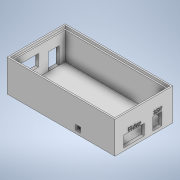
# Autodesk Inventor part: Caixa plaquinha valvula
Saved by Autodesk Inventor 2020 (Build 240168000, 168)
## iProperties
Created: 2022-10-16
Part Number: Caixa plaquinha valvula
Material: Genérico
Document SubType Name: Modeling
Designer: Gabriel
Density: 1 g/cm^3
Appearance: Padrão
Author: Gabriel
Autodesk Inventor part; units mm, degrees
ref_plane "YZ Plane" through (0, 0, 0) normal (1, 0, 0) x (0, 1, 0)
ref_plane "XZ Plane" through (0, 0, 0) normal (0, 1, 0) x (-1, 0, 0)
ref_plane "XY Plane" through (0, 0, 0) normal (0, 0, 1) x (1, 0, 0)
sketch "Esboço1" plane through (0, 0, 0) normal (0, 1, 0) x (-1, 0, 0)
  line L0 (62.5795, 27.2159) -> (-45.4205, 27.2159)
  line L1 (-45.4205, 27.2159) -> (-45.4205, -30.7841)
  line L2 (-45.4205, -30.7841) -> (62.5795, -30.7841)
  line L3 (62.5795, -30.7841) -> (62.5795, 27.2159)
  point P0 (0, 0)
  dimension "d0" = 58
  dimension "d1" = 108
  constraints: 8 end point, 2 parallel, 1 horizontal, 1 perpendicular
  measures "d0" distance between parallel lines of L2 L0
  measures "d1" distance of L1.end L2.end
extrude "Extrusão1" add sketch "Esboço1" along normal blind 32
sketch "Esboço2" plane through (0, 32, 0) normal (0, 1, 0) x (1, 0, 0)
  line L0 (-59.5795, 27.7841) -> (42.4205, 27.7841)
  line L1 (42.4205, 27.7841) -> (42.4205, -24.2159)
  line L2 (42.4205, -24.2159) -> (-59.5795, -24.2159)
  line L3 (-59.5795, -24.2159) -> (-59.5795, 27.7841)
  line L4 (-62.5795, 30.7841) -> (-62.5795, -27.2159) projected
  line L5 (45.4205, 30.7841) -> (-62.5795, 30.7841) projected
  point P0 (0, 0)
  dimension "d4" = 3
  dimension "d5" = 102
  dimension "d6" = 3
  dimension "d7" = 52
  constraints: 8 end point, 2 parallel, 1 horizontal, 1 perpendicular
  measures "d4" distance between parallel lines of L4 L3
  measures "d5" distance between parallel lines of L1 L3
  measures "d6" distance between parallel lines of L5 L0
  measures "d7" distance between parallel lines of L0 L2
extrude "Extrusão2" cut sketch "Esboço2" against normal blind 30
sketch "Esboço4" plane through (0, 32, 0) normal (0, 1, 0) x (1, 0, 0)
  line L0 (-61.0795, 29.2841) -> (43.9205, 29.2841)
  line L1 (43.9205, 29.2841) -> (43.9205, -25.7159)
  line L2 (43.9205, -25.7159) -> (-61.0795, -25.7159)
  line L3 (-61.0795, -25.7159) -> (-61.0795, 29.2841)
  line L4 (45.4205, 30.7841) -> (-62.5795, 30.7841) projected
  line L5 (-62.5795, 30.7841) -> (-62.5795, -27.2159) projected
  line L6 (-62.5795, -27.2159) -> (45.4205, -27.2159) projected
  line L7 (45.4205, -27.2159) -> (45.4205, 30.7841) projected
  point P0 (0, 0)
  dimension "d10" = 1.5
  dimension "d11" = 1.5
  dimension "d12" = 1.5
  dimension "d13" = 1.5
  constraints: 8 end point, 2 parallel, 1 horizontal, 1 perpendicular
  measures "d10" distance between parallel lines of L4 L0
  measures "d11" distance between parallel lines of L5 L3
  measures "d12" distance between parallel lines of L6 L2
  measures "d13" distance between parallel lines of L7 L1
extrude "Extrusão3" cut sketch "Esboço4" against normal blind 2.5 contours L0 L1 L2 L3
sketch "Esboço5" plane through (42.4205, 2, -27.7841) normal (-1, 0, 0) x (0, 0, 1)
  line L0 (0, 0) -> (52, 0) projected
  line L1 (8.1, 0) -> (17.1, 0)
  line L2 (17.1, 0) -> (17.1, 13.5)
  line L3 (17.1, 13.5) -> (8.1, 13.5)
  line L4 (8.1, 13.5) -> (8.1, 0)
  line L5 (46.3, 0) -> (25.6, 0)
  line L6 (25.6, 0) -> (25.6, 12)
  line L7 (25.6, 12) -> (46.3, 12)
  line L8 (46.3, 12) -> (46.3, 0)
  line L9 (52, 27.5) -> (0, 27.5) projected
  point P0 (27.7841, -2)
  point P1 (25.6, 0)
  point P2 (17.1, 0)
  dimension "d17" = 9
  dimension "d18" = 13.5
  dimension "d20" = 20.7
  dimension "d21" = 12
  dimension "d23" = 8.5
  dimension "d24" = 8.1
  dimension "d25" = 5.7
  dimension "d28" = 15.5
  constraints: 16 end point, 4 parallel, 2 horizontal, 2 perpendicular, 2 point on line
  measures "d17" distance between parallel lines of L2 L4
  measures "d18" distance between parallel lines of L0 L3
  measures "d20" distance between parallel lines of L6 L8
  measures "d21" distance between parallel lines of L0 L7
  measures "d23" distance between parallel lines of L6 L2
  measures "d24" distance from line of L9.end L4
  measures "d25" distance from line of L9.start L8
  measures "d28" distance between parallel lines of L9 L7
extrude "Extrusão4" cut sketch "Esboço5" against normal blind 5
sketch "Esboço6" plane through (0, 2, 0) normal (0, 1, 0) x (1, 0, 0)
  line L0 (45.4205, 2.1841) -> (45.4205, -18.5159) projected
  line L1 (42.4205, 10.6841) -> (42.4205, 2.1841) projected
  line L2 (45.4205, -18.5159) -> (42.4205, -18.5159)
  line L3 (42.4205, -18.5159) -> (42.4205, 2.1841)
  line L4 (42.4205, 2.1841) -> (45.4205, 2.1841)
  line L5 (45.4205, 2.1841) -> (45.4205, -18.5159)
  line L6 (45.4205, 19.6841) -> (45.4205, 10.6841) projected
  line L7 (45.4205, 19.6841) -> (42.4205, 19.6841)
  line L8 (42.4205, 19.6841) -> (42.4205, 10.6841)
  line L9 (42.4205, 10.6841) -> (45.4205, 10.6841)
  line L10 (45.4205, 10.6841) -> (45.4205, 19.6841)
  point P0 (0, 0)
  constraints: 16 end point, 4 parallel, 2 horizontal, 2 perpendicular, 1 point on line
extrude "Extrusão5" add sketch "Esboço6" along normal blind 1
sketch "Esboço7" plane through (-59.5795, 2, 24.2159) normal (1, 0, 0) x (0, 0, -1)
  line L0 (46, 0.1025) -> (35, 0.1025)
  line L1 (35, 0.1025) -> (35, 17.0506)
  line L2 (35, 17.0506) -> (46, 17.0506)
  line L3 (46, 17.0506) -> (46, 0.1025)
  line L4 (3.908, 8.6) -> (25.408, 8.6)
  line L5 (25.408, 8.6) -> (25.408, 20.6)
  line L6 (25.408, 20.6) -> (3.908, 20.6)
  line L7 (3.908, 20.6) -> (3.908, 8.6)
  line L8 (0, 0) -> (52, 0) projected
  point P0 (24.2159, -2)
  point P1 (52, 27.5)
  point P2 (0, 27.5)
  dimension "d31" = 6
  dimension "d32" = 11
  dimension "d33" = 3.908
  dimension "d34" = 21.5
  dimension "d35" = 12
  dimension "d36" = 8.6
  dimension "d39" = 16.948
  constraints: 16 end point, 4 parallel, 2 horizontal, 2 perpendicular
  measures "d31" distance from line of L3 point (52, 27.5)
  measures "d32" distance between parallel lines of L3 L1
  measures "d33" distance from line of point (0, 27.5) L7
  measures "d34" distance between parallel lines of L5 L7
  measures "d35" distance between parallel lines of L6 L4
  measures "d36" distance between parallel lines of L8 L4
  measures "d39" distance between parallel lines of L0 L2
extrude "Extrusão6" cut sketch "Esboço7" against normal blind 5
sketch "Esboço8" plane through (42.4205, 2, 24.2159) normal (0, 0, -1) x (-1, 0, 0)
  line L0 (0, 0) -> (102, 0) projected
  line L1 (36.5, 0) -> (31.5, 0)
  line L2 (31.5, 0) -> (31.5, 6)
  line L3 (31.5, 6) -> (36.5, 6)
  line L4 (36.5, 6) -> (36.5, 0)
  line L5 (0, 27.5) -> (0, 0) projected
  point P0 (42.4205, -2)
  dimension "d41" = 5
  dimension "d43" = 31.5
  dimension "d44" = 6
  dimension "d45" = 6
  constraints: 8 end point, 2 parallel, 1 horizontal, 1 perpendicular, 1 point on line
  measures "d41" distance between parallel lines of L4 L2
  measures "d43" distance between parallel lines of L5 L2
  measures "d44" distance between parallel lines of L3 L1
  measures "d45" distance between parallel lines of L0 L3
extrude "Extrusão7" cut sketch "Esboço8" against normal blind 5
sketch "Esboço9" plane through (0, 2, 0) normal (0, 1, 0) x (1, 0, 0)
  line L0 (5.9205, -24.2159) -> (-59.5795, -24.2159) projected
  line L1 (5.9205, -24.2159) -> (10.9205, -24.2159)
  line L2 (10.9205, -24.2159) -> (10.9205, -27.2159)
  line L3 (10.9205, -27.2159) -> (5.9205, -27.2159)
  line L4 (5.9205, -27.2159) -> (5.9205, -24.2159)
  line L5 (10.9205, -27.2159) -> (5.9205, -27.2159) projected
  point P0 (0, 0)
  dimension "d50" = 0
  constraints: 8 end point, 2 parallel, 1 horizontal, 1 perpendicular
  measures "d50" distance between parallel lines of L5 L3
extrude "Extrusão8" add sketch "Esboço9" along normal blind 1
sketch "Esboço10" plane through (45.4205, 0, 27.2159) normal (1, 0, 0) x (0, 0, -1)
  line L0 (36.0799, 21.9524) -> (48.8276, 21.9524) construction
  line L1 (48.8276, 21.9524) -> (48.8276, 15.4026) construction
  line L2 (48.8276, 15.4026) -> (36.0799, 15.4026) construction
  line L3 (36.0799, 15.4026) -> (36.0799, 21.9524) construction
  line L4 (13.7499, 18.2381) -> (24.4451, 18.2381) construction
  line L5 (24.4451, 18.2381) -> (24.4451, 15.1259) construction
  line L6 (24.4451, 15.1259) -> (13.7499, 15.1259) construction
  line L7 (13.7499, 15.1259) -> (13.7499, 18.2381) construction
  line L8 (16.286, 15.1881) -> (15.5247, 15.1881)
  line L9 (15.5247, 15.1881) -> (15.5247, 17.2099)
  line L10 (15.5247, 17.2099) -> (14.9711, 15.9049)
  line L11 (14.9711, 15.9049) -> (14.4471, 15.9049)
  line L12 (14.4471, 15.9049) -> (13.8935, 17.2099)
  line L13 (13.8935, 17.2099) -> (13.8935, 15.1881)
  line L14 (13.8935, 15.1881) -> (13.1717, 15.1881)
  line L15 (13.1717, 15.1881) -> (13.1717, 18.2381)
  line L16 (13.1717, 18.2381) -> (14.0541, 18.2381)
  line L17 (14.0541, 18.2381) -> (14.7313, 16.7329)
  line L18 (14.7313, 16.7329) -> (15.4036, 18.2381)
  line L19 (15.4036, 18.2381) -> (16.286, 18.2381)
  line L20 (16.286, 18.2381) -> (16.286, 15.1881)
  spline S0 degree 2 poles (19.0839, 16.3374) (19.0839, 15.769) (18.4635, 15.1165) (17.8975, 15.1165) knots 0 0 0 1 2 2 2
  spline S1 degree 2 poles (17.8975, 15.1165) (17.334, 15.1165) (16.7087, 15.769) (16.7087, 16.3374) knots 0 0 0 1 2 2 2
  spline S2 degree 2 poles (16.7087, 16.3374) (16.7087, 16.9109) (17.334, 17.5609) (17.8975, 17.5609) knots 0 0 0 1 2 2 2
  spline S3 degree 2 poles (17.8975, 17.5609) (18.461, 17.5609) (19.0839, 16.9084) (19.0839, 16.3374) knots 0 0 0 1 2 2 2
  spline S4 degree 2 poles (18.3498, 16.3325) (18.3498, 16.5376) (18.2831, 16.812) (18.2238, 16.8936) knots 0 0 0 1 2 2 2
  spline S5 degree 2 poles (18.2238, 16.8936) (18.1595, 16.9801) (17.9989, 17.0468) (17.8975, 17.0468) knots 0 0 0 1 2 2 2
  spline S6 degree 2 poles (17.8975, 17.0468) (17.7986, 17.0468) (17.6429, 16.9875) (17.5787, 16.9034) knots 0 0 0 1 2 2 2
  spline S7 degree 2 poles (17.5787, 16.9034) (17.5169, 16.8244) (17.4427, 16.5451) (17.4427, 16.3325) knots 0 0 0 1 2 2 2
  spline S8 degree 2 poles (17.4427, 16.3325) (17.4427, 16.1224) (17.5119, 15.8629) (17.5688, 15.7838) knots 0 0 0 1 2 2 2
  spline S9 degree 2 poles (17.5688, 15.7838) (17.6256, 15.7047) (17.7986, 15.6306) (17.9025, 15.6306) knots 0 0 0 1 2 2 2
  spline S10 degree 2 poles (17.9025, 15.6306) (17.989, 15.6306) (18.1669, 15.7047) (18.2213, 15.7789) knots 0 0 0 1 2 2 2
  spline S11 degree 2 poles (18.2213, 15.7789) (18.2831, 15.8654) (18.3498, 16.115) (18.3498, 16.3325) knots 0 0 0 1 2 2 2
  spline S12 degree 2 poles (20.3444, 15.1436) (19.907, 15.1436) (19.5065, 15.5045) (19.5065, 15.9148) knots 0 0 0 1 2 2 2
  line L21 (19.5065, 15.9148) -> (19.5065, 16.99)
  line L22 (19.5065, 16.99) -> (19.2322, 16.99)
  line L23 (19.2322, 16.99) -> (19.2322, 17.4892)
  line L24 (19.2322, 17.4892) -> (19.5065, 17.4892)
  line L25 (19.5065, 17.4892) -> (19.5065, 18.1467)
  line L26 (19.5065, 18.1467) -> (20.2233, 18.1467)
  line L27 (20.2233, 18.1467) -> (20.2233, 17.4892)
  line L28 (20.2233, 17.4892) -> (20.9154, 17.4892)
  line L29 (20.9154, 17.4892) -> (20.9154, 16.99)
  line L30 (20.9154, 16.99) -> (20.2233, 16.99)
  line L31 (20.2233, 16.99) -> (20.2233, 16.1718)
  spline S13 degree 2 poles (20.2233, 16.1718) (20.2233, 16.0507) (20.2283, 15.8703) (20.2579, 15.7986) knots 0 0 0 1 2 2 2
  spline S14 degree 2 poles (20.2579, 15.7986) (20.2876, 15.7269) (20.4334, 15.6429) (20.5718, 15.6429) knots 0 0 0 1 2 2 2
  spline S15 degree 2 poles (20.5718, 15.6429) (20.6311, 15.6429) (20.8165, 15.6923) (20.8536, 15.7121) knots 0 0 0 1 2 2 2
  line L32 (20.8536, 15.7121) -> (20.9154, 15.7121)
  line L33 (20.9154, 15.7121) -> (20.9154, 15.2079)
  spline S16 degree 2 poles (20.9154, 15.2079) (20.7992, 15.1782) (20.5372, 15.1436) (20.3444, 15.1436) knots 0 0 0 1 2 2 2
  spline S17 degree 2 poles (23.4142, 16.3374) (23.4142, 15.769) (22.7938, 15.1165) (22.2278, 15.1165) knots 0 0 0 1 2 2 2
  spline S18 degree 2 poles (22.2278, 15.1165) (21.6643, 15.1165) (21.039, 15.769) (21.039, 16.3374) knots 0 0 0 1 2 2 2
  spline S19 degree 2 poles (21.039, 16.3374) (21.039, 16.9109) (21.6643, 17.5609) (22.2278, 17.5609) knots 0 0 0 1 2 2 2
  spline S20 degree 2 poles (22.2278, 17.5609) (22.7914, 17.5609) (23.4142, 16.9084) (23.4142, 16.3374) knots 0 0 0 1 2 2 2
  spline S21 degree 2 poles (22.6801, 16.3325) (22.6801, 16.5376) (22.6134, 16.812) (22.5541, 16.8936) knots 0 0 0 1 2 2 2
  spline S22 degree 2 poles (22.5541, 16.8936) (22.4898, 16.9801) (22.3292, 17.0468) (22.2278, 17.0468) knots 0 0 0 1 2 2 2
  spline S23 degree 2 poles (22.2278, 17.0468) (22.129, 17.0468) (21.9732, 16.9875) (21.909, 16.9034) knots 0 0 0 1 2 2 2
  spline S24 degree 2 poles (21.909, 16.9034) (21.8472, 16.8244) (21.773, 16.5451) (21.773, 16.3325) knots 0 0 0 1 2 2 2
  spline S25 degree 2 poles (21.773, 16.3325) (21.773, 16.1224) (21.8422, 15.8629) (21.8991, 15.7838) knots 0 0 0 1 2 2 2
  spline S26 degree 2 poles (21.8991, 15.7838) (21.9559, 15.7047) (22.129, 15.6306) (22.2328, 15.6306) knots 0 0 0 1 2 2 2
  spline S27 degree 2 poles (22.2328, 15.6306) (22.3193, 15.6306) (22.4972, 15.7047) (22.5516, 15.7789) knots 0 0 0 1 2 2 2
  spline S28 degree 2 poles (22.5516, 15.7789) (22.6134, 15.8654) (22.6801, 16.115) (22.6801, 16.3325) knots 0 0 0 1 2 2 2
  line L34 (25.3396, 16.8095) -> (25.2803, 16.8095)
  spline S29 degree 2 poles (25.2803, 16.8095) (25.2383, 16.8244) (25.0826, 16.8392) (24.9886, 16.8392) knots 0 0 0 1 2 2 2
  spline S30 degree 2 poles (24.9886, 16.8392) (24.8774, 16.8392) (24.6278, 16.7725) (24.5116, 16.728) knots 0 0 0 1 2 2 2
  line L35 (24.5116, 16.728) -> (24.5116, 15.1881)
  line L36 (24.5116, 15.1881) -> (23.7948, 15.1881)
  line L37 (23.7948, 15.1881) -> (23.7948, 17.4892)
  line L38 (23.7948, 17.4892) -> (24.5116, 17.4892)
  line L39 (24.5116, 17.4892) -> (24.5116, 17.158)
  spline S31 degree 2 poles (24.5116, 17.158) (24.561, 17.2025) (24.7341, 17.3409) (24.8057, 17.3829) knots 0 0 0 1 2 2 2
  spline S32 degree 2 poles (24.8057, 17.3829) (24.8848, 17.4299) (25.0924, 17.4966) (25.1839, 17.4966) knots 0 0 0 1 2 2 2
  spline S33 degree 2 poles (25.1839, 17.4966) (25.2185, 17.4966) (25.305, 17.4917) (25.3396, 17.4892) knots 0 0 0 1 2 2 2
  line L40 (25.3396, 17.4892) -> (25.3396, 16.8095)
  line L41 (40.7496, 17.1229) -> (38.7352, 17.1229)
  line L42 (38.7352, 17.1229) -> (38.7352, 17.6543)
  line L43 (38.7352, 17.6543) -> (39.3778, 17.6543)
  line L44 (39.3778, 17.6543) -> (39.3778, 19.2683)
  line L45 (39.3778, 19.2683) -> (38.7352, 19.2683)
  line L46 (38.7352, 19.2683) -> (38.7352, 19.7651)
  spline S34 degree 2 poles (38.7352, 19.7651) (38.8761, 19.7651) (39.1554, 19.8021) (39.2394, 19.8417) knots 0 0 0 1 2 2 2
  spline S35 degree 2 poles (39.2394, 19.8417) (39.3358, 19.8911) (39.4445, 20.0567) (39.4544, 20.1803) knots 0 0 0 1 2 2 2
  line L47 (39.4544, 20.1803) -> (40.1218, 20.1803)
  line L48 (40.1218, 20.1803) -> (40.1218, 17.6543)
  line L49 (40.1218, 17.6543) -> (40.7496, 17.6543)
  line L50 (40.7496, 17.6543) -> (40.7496, 17.1229)
  line L51 (43.5573, 17.1229) -> (41.3156, 17.1229)
  line L52 (41.3156, 17.1229) -> (41.3156, 17.6197)
  spline S36 degree 2 poles (41.3156, 17.6197) (41.5998, 17.8471) (42.0546, 18.2475) (42.2251, 18.4279) knots 0 0 0 1 2 2 2
  spline S37 degree 2 poles (42.2251, 18.4279) (42.45, 18.6627) (42.6502, 19.0211) (42.6502, 19.2089) knots 0 0 0 1 2 2 2
  spline S38 degree 2 poles (42.6502, 19.2089) (42.6502, 19.4215) (42.3957, 19.6489) (42.1683, 19.6489) knots 0 0 0 1 2 2 2
  spline S39 degree 2 poles (42.1683, 19.6489) (42.0521, 19.6489) (41.8445, 19.592) (41.7382, 19.5476) knots 0 0 0 1 2 2 2
  spline S40 degree 2 poles (41.7382, 19.5476) (41.6344, 19.5006) (41.4861, 19.4017) (41.449, 19.377) knots 0 0 0 1 2 2 2
  line L53 (41.449, 19.377) -> (41.3897, 19.377)
  line L54 (41.3897, 19.377) -> (41.3897, 20.0419)
  spline S41 degree 2 poles (41.3897, 20.0419) (41.5182, 20.1037) (42.0669, 20.2322) (42.3215, 20.2322) knots 0 0 0 1 2 2 2
  spline S42 degree 2 poles (42.3215, 20.2322) (42.8653, 20.2322) (43.4239, 19.7478) (43.4239, 19.3103) knots 0 0 0 1 2 2 2
  spline S43 degree 2 poles (43.4239, 19.3103) (43.4239, 19.0409) (43.1693, 18.5218) (42.8752, 18.2252) knots 0 0 0 1 2 2 2
  spline S44 degree 2 poles (42.8752, 18.2252) (42.6898, 18.0423) (42.3413, 17.7581) (42.2647, 17.6988) knots 0 0 0 1 2 2 2
  line L55 (42.2647, 17.6988) -> (43.5573, 17.6988)
  line L56 (43.5573, 17.6988) -> (43.5573, 17.1229)
  line L57 (46.5406, 20.1729) -> (45.4926, 17.1229)
  line L58 (45.4926, 17.1229) -> (44.6943, 17.1229)
  line L59 (44.6943, 17.1229) -> (43.6463, 20.1729)
  line L60 (43.6463, 20.1729) -> (44.4397, 20.1729)
  line L61 (44.4397, 20.1729) -> (45.1046, 18.1041)
  line L62 (45.1046, 18.1041) -> (45.767, 20.1729)
  line L63 (45.767, 20.1729) -> (46.5406, 20.1729)
  point P0 (27.2159, 0)
  constraints: 4 other
extrude "Extrusão9" add sketch "Esboço10" along normal blind 0.8
sketch "Esboço11" plane through (-62.5795, 0, -30.7841) normal (-1, 0, 0) x (0, 0, 1)
  line L0 (35.5434, 8.3072) -> (44.2454, 8.3072) construction
  line L1 (44.2454, 8.3072) -> (44.2454, 5.1577) construction
  line L2 (44.2454, 5.1577) -> (35.5434, 5.1577) construction
  line L3 (35.5434, 5.1577) -> (35.5434, 8.3072) construction
  line L4 (8.7914, 24.4501) -> (20.5601, 24.4501) construction
  line L5 (20.5601, 24.4501) -> (20.5601, 20.4793) construction
  line L6 (20.5601, 20.4793) -> (8.7914, 20.4793) construction
  line L7 (8.7914, 20.4793) -> (8.7914, 24.4501) construction
  spline S0 degree 2 poles (10.2203, 22.2218) (10.2203, 21.7711) (9.4559, 21.2084) (8.8011, 21.2084) knots 0 0 0 1 2 2 2
  spline S1 degree 2 poles (8.8011, 21.2084) (8.4226, 21.2084) (7.8599, 21.3404) (7.6135, 21.4449) knots 0 0 0 1 2 2 2
  line L8 (7.6135, 21.4449) -> (7.6135, 22.1745)
  line L9 (7.6135, 22.1745) -> (7.7006, 22.1745)
  spline S2 degree 2 poles (7.7006, 22.1745) (7.9421, 21.9803) (8.5471, 21.7711) (8.826, 21.7711) knots 0 0 0 1 2 2 2
  spline S3 degree 2 poles (8.826, 21.7711) (8.8982, 21.7711) (9.1297, 21.796) (9.2044, 21.8234) knots 0 0 0 1 2 2 2
  spline S4 degree 2 poles (9.2044, 21.8234) (9.2941, 21.8607) (9.4111, 21.9728) (9.4111, 22.0798) knots 0 0 0 1 2 2 2
  spline S5 degree 2 poles (9.4111, 22.0798) (9.4111, 22.1819) (9.2418, 22.3263) (9.0775, 22.3662) knots 0 0 0 1 2 2 2
  spline S6 degree 2 poles (9.0775, 22.3662) (8.9057, 22.406) (8.5222, 22.4782) (8.3529, 22.533) knots 0 0 0 1 2 2 2
  spline S7 degree 2 poles (8.3529, 22.533) (7.9695, 22.6575) (7.6309, 23.0857) (7.6309, 23.4044) knots 0 0 0 1 2 2 2
  spline S8 degree 2 poles (7.6309, 23.4044) (7.6309, 23.8302) (8.3953, 24.368) (8.9953, 24.368) knots 0 0 0 1 2 2 2
  spline S9 degree 2 poles (8.9953, 24.368) (9.2966, 24.368) (9.8842, 24.2509) (10.0983, 24.1638) knots 0 0 0 1 2 2 2
  line L10 (10.0983, 24.1638) -> (10.0983, 23.4617)
  line L11 (10.0983, 23.4617) -> (10.0136, 23.4617)
  spline S10 degree 2 poles (10.0136, 23.4617) (9.8294, 23.6086) (9.2966, 23.8078) (9.0177, 23.8078) knots 0 0 0 1 2 2 2
  spline S11 degree 2 poles (9.0177, 23.8078) (8.9181, 23.8078) (8.7239, 23.7804) (8.6343, 23.743) knots 0 0 0 1 2 2 2
  spline S12 degree 2 poles (8.6343, 23.743) (8.5546, 23.7132) (8.4401, 23.5887) (8.4401, 23.509) knots 0 0 0 1 2 2 2
  spline S13 degree 2 poles (8.4401, 23.509) (8.4401, 23.387) (8.6243, 23.2575) (8.8808, 23.2052) knots 0 0 0 1 2 2 2
  spline S14 degree 2 poles (8.8808, 23.2052) (9.0476, 23.1704) (9.3588, 23.1056) (9.5356, 23.0484) knots 0 0 0 1 2 2 2
  spline S15 degree 2 poles (9.5356, 23.0484) (9.8866, 22.9314) (10.2203, 22.538) (10.2203, 22.2218) knots 0 0 0 1 2 2 2
  line L12 (11.4577, 21.2632) -> (10.7182, 21.2632)
  line L13 (10.7182, 21.2632) -> (10.7182, 23.5638)
  line L14 (10.7182, 23.5638) -> (11.4577, 23.5638)
  line L15 (11.4577, 23.5638) -> (11.4577, 21.2632)
  line L16 (11.4776, 23.8899) -> (10.6983, 23.8899)
  line L17 (10.6983, 23.8899) -> (10.6983, 24.4501)
  line L18 (10.6983, 24.4501) -> (11.4776, 24.4501)
  line L19 (11.4776, 24.4501) -> (11.4776, 23.8899)
  spline S16 degree 2 poles (14.3882, 21.5271) (14.3882, 21.2034) (14.2039, 20.7603) (14.0371, 20.6358) knots 0 0 0 1 2 2 2
  spline S17 degree 2 poles (14.0371, 20.6358) (13.8728, 20.5088) (13.4047, 20.3967) (13.1084, 20.3967) knots 0 0 0 1 2 2 2
  spline S18 degree 2 poles (13.1084, 20.3967) (12.8694, 20.3967) (12.4038, 20.454) (12.2345, 20.4963) knots 0 0 0 1 2 2 2
  line L20 (12.2345, 20.4963) -> (12.2345, 21.0715)
  line L21 (12.2345, 21.0715) -> (12.3242, 21.0715)
  spline S19 degree 2 poles (12.3242, 21.0715) (12.4586, 21.0192) (12.847, 20.9296) (13.0014, 20.9296) knots 0 0 0 1 2 2 2
  spline S20 degree 2 poles (13.0014, 20.9296) (13.2055, 20.9296) (13.4595, 21.0043) (13.5292, 21.074) knots 0 0 0 1 2 2 2
  spline S21 degree 2 poles (13.5292, 21.074) (13.5915, 21.1412) (13.6487, 21.3454) (13.6487, 21.4873) knots 0 0 0 1 2 2 2
  line L22 (13.6487, 21.4873) -> (13.6487, 21.5321)
  spline S22 degree 2 poles (13.6487, 21.5321) (13.5168, 21.4225) (13.1931, 21.2956) (12.9939, 21.2956) knots 0 0 0 1 2 2 2
  spline S23 degree 2 poles (12.9939, 21.2956) (12.5109, 21.2956) (11.988, 21.8782) (11.988, 22.4707) knots 0 0 0 1 2 2 2
  spline S24 degree 2 poles (11.988, 22.4707) (11.988, 22.7546) (12.1474, 23.1704) (12.2918, 23.3223) knots 0 0 0 1 2 2 2
  spline S25 degree 2 poles (12.2918, 23.3223) (12.4287, 23.4667) (12.8221, 23.626) (13.0288, 23.626) knots 0 0 0 1 2 2 2
  spline S26 degree 2 poles (13.0288, 23.626) (13.2155, 23.626) (13.5193, 23.5389) (13.6437, 23.4592) knots 0 0 0 1 2 2 2
  line L23 (13.6437, 23.4592) -> (13.6711, 23.5638)
  line L24 (13.6711, 23.5638) -> (14.3882, 23.5638)
  line L25 (14.3882, 23.5638) -> (14.3882, 21.5271)
  line L26 (13.6487, 21.9877) -> (13.6487, 23.0309)
  spline S27 degree 2 poles (13.6487, 23.0309) (13.5865, 23.0583) (13.4022, 23.0882) (13.3275, 23.0882) knots 0 0 0 1 2 2 2
  spline S28 degree 2 poles (13.3275, 23.0882) (13.0387, 23.0882) (12.7474, 22.7546) (12.7474, 22.4558) knots 0 0 0 1 2 2 2
  spline S29 degree 2 poles (12.7474, 22.4558) (12.7474, 22.1222) (12.9939, 21.8607) (13.2379, 21.8607) knots 0 0 0 1 2 2 2
  spline S30 degree 2 poles (13.2379, 21.8607) (13.3475, 21.8607) (13.5616, 21.9305) (13.6487, 21.9877) knots 0 0 0 1 2 2 2
  line L27 (17.3959, 21.2632) -> (16.6564, 21.2632)
  line L28 (16.6564, 21.2632) -> (16.6564, 22.4035)
  spline S31 degree 2 poles (16.6564, 22.4035) (16.6564, 22.5429) (16.6265, 22.8193) (16.5942, 22.8865) knots 0 0 0 1 2 2 2
  spline S32 degree 2 poles (16.5942, 22.8865) (16.5518, 22.9612) (16.395, 23.0309) (16.253, 23.0309) knots 0 0 0 1 2 2 2
  spline S33 degree 2 poles (16.253, 23.0309) (16.1535, 23.0309) (15.9468, 22.9662) (15.8248, 22.894) knots 0 0 0 1 2 2 2
  line L29 (15.8248, 22.894) -> (15.8248, 21.2632)
  line L30 (15.8248, 21.2632) -> (15.0853, 21.2632)
  line L31 (15.0853, 21.2632) -> (15.0853, 23.5638)
  line L32 (15.0853, 23.5638) -> (15.8248, 23.5638)
  line L33 (15.8248, 23.5638) -> (15.8248, 23.3098)
  spline S34 degree 2 poles (15.8248, 23.3098) (16.0215, 23.4617) (16.3825, 23.626) (16.6041, 23.626) knots 0 0 0 1 2 2 2
  spline S35 degree 2 poles (16.6041, 23.626) (16.9776, 23.626) (17.3959, 23.1928) (17.3959, 22.7596) knots 0 0 0 1 2 2 2
  line L34 (17.3959, 22.7596) -> (17.3959, 21.2632)
  spline S36 degree 2 poles (19.4674, 21.5072) (19.4076, 21.4624) (19.2308, 21.3354) (19.1537, 21.2981) knots 0 0 0 1 2 2 2
  spline S37 degree 2 poles (19.1537, 21.2981) (19.0441, 21.2483) (18.8126, 21.2009) (18.6731, 21.2009) knots 0 0 0 1 2 2 2
  spline S38 degree 2 poles (18.6731, 21.2009) (18.3445, 21.2009) (17.9013, 21.6068) (17.9013, 21.923) knots 0 0 0 1 2 2 2
  spline S39 degree 2 poles (17.9013, 21.923) (17.9013, 22.1745) (18.1279, 22.4932) (18.3345, 22.5853) knots 0 0 0 1 2 2 2
  spline S40 degree 2 poles (18.3345, 22.5853) (18.5387, 22.6774) (19.1462, 22.7571) (19.4724, 22.7745) knots 0 0 0 1 2 2 2
  line L35 (19.4724, 22.7745) -> (19.4724, 22.7869)
  spline S41 degree 2 poles (19.4724, 22.7869) (19.4724, 22.9787) (19.1611, 23.1231) (18.8574, 23.1231) knots 0 0 0 1 2 2 2
  spline S42 degree 2 poles (18.8574, 23.1231) (18.6756, 23.1231) (18.2598, 22.9936) (18.1702, 22.9587) knots 0 0 0 1 2 2 2
  line L36 (18.1702, 22.9587) -> (18.103, 22.9587)
  line L37 (18.103, 22.9587) -> (18.103, 23.514)
  spline S43 degree 2 poles (18.103, 23.514) (18.22, 23.5438) (18.7453, 23.6285) (19.0117, 23.6285) knots 0 0 0 1 2 2 2
  spline S44 degree 2 poles (19.0117, 23.6285) (19.6392, 23.6285) (20.1994, 23.2426) (20.1994, 22.8268) knots 0 0 0 1 2 2 2
  line L38 (20.1994, 22.8268) -> (20.1994, 21.2632)
  line L39 (20.1994, 21.2632) -> (19.4674, 21.2632)
  line L40 (19.4674, 21.2632) -> (19.4674, 21.5072)
  line L41 (19.4674, 21.8632) -> (19.4674, 22.3413)
  spline S45 degree 2 poles (19.4674, 22.3413) (19.318, 22.3288) (18.9694, 22.2865) (18.8773, 22.2566) knots 0 0 0 1 2 2 2
  spline S46 degree 2 poles (18.8773, 22.2566) (18.7677, 22.2243) (18.6507, 22.0898) (18.6507, 21.9827) knots 0 0 0 1 2 2 2
  spline S47 degree 2 poles (18.6507, 21.9827) (18.6507, 21.9105) (18.6756, 21.8209) (18.7254, 21.7811) knots 0 0 0 1 2 2 2
  spline S48 degree 2 poles (18.7254, 21.7811) (18.7727, 21.7412) (18.9022, 21.7014) (19.0416, 21.7014) knots 0 0 0 1 2 2 2
  spline S49 degree 2 poles (19.0416, 21.7014) (19.1537, 21.7014) (19.3802, 21.791) (19.4674, 21.8632) knots 0 0 0 1 2 2 2
  line L42 (21.6161, 21.2632) -> (20.8766, 21.2632)
  line L43 (20.8766, 21.2632) -> (20.8766, 24.4501)
  line L44 (20.8766, 24.4501) -> (21.6161, 24.4501)
  line L45 (21.6161, 24.4501) -> (21.6161, 21.2632)
  spline S50 degree 2 poles (37.1274, 5.1386) (36.5119, 5.1386) (35.8495, 5.7318) (35.8495, 6.3052) knots 0 0 0 1 2 2 2
  line L46 (35.8495, 6.3052) -> (35.8495, 8.2529)
  line L47 (35.8495, 8.2529) -> (36.6158, 8.2529)
  line L48 (36.6158, 8.2529) -> (36.6158, 6.3497)
  spline S51 degree 2 poles (36.6158, 6.3497) (36.6158, 6.0309) (36.8555, 5.7194) (37.1274, 5.7194) knots 0 0 0 1 2 2 2
  spline S52 degree 2 poles (37.1274, 5.7194) (37.3919, 5.7194) (37.639, 6.0185) (37.639, 6.3497) knots 0 0 0 1 2 2 2
  line L49 (37.639, 6.3497) -> (37.639, 8.2529)
  line L50 (37.639, 8.2529) -> (38.4052, 8.2529)
  line L51 (38.4052, 8.2529) -> (38.4052, 6.3077)
  spline S53 degree 2 poles (38.4052, 6.3077) (38.4052, 5.7442) (37.7601, 5.1386) (37.1274, 5.1386) knots 0 0 0 1 2 2 2
  spline S54 degree 2 poles (39.9352, 5.1485) (39.5842, 5.1485) (39.0553, 5.2844) (38.8279, 5.3833) knots 0 0 0 1 2 2 2
  line L52 (38.8279, 5.3833) -> (38.8279, 6.11)
  line L53 (38.8279, 6.11) -> (38.8971, 6.11)
  spline S55 degree 2 poles (38.8971, 6.11) (39.1269, 5.9147) (39.6781, 5.7046) (39.9376, 5.7046) knots 0 0 0 1 2 2 2
  spline S56 degree 2 poles (39.9376, 5.7046) (40.0044, 5.7046) (40.2194, 5.7343) (40.2837, 5.7639) knots 0 0 0 1 2 2 2
  spline S57 degree 2 poles (40.2837, 5.7639) (40.3628, 5.7985) (40.474, 5.9246) (40.474, 6.0259) knots 0 0 0 1 2 2 2
  spline S58 degree 2 poles (40.474, 6.0259) (40.474, 6.1421) (40.2936, 6.2854) (40.17, 6.3176) knots 0 0 0 1 2 2 2
  spline S59 degree 2 poles (40.17, 6.3176) (40.0143, 6.3596) (39.6608, 6.4313) (39.5051, 6.4856) knots 0 0 0 1 2 2 2
  spline S60 degree 2 poles (39.5051, 6.4856) (39.1517, 6.6092) (38.8452, 7.0319) (38.8452, 7.3482) knots 0 0 0 1 2 2 2
  spline S61 degree 2 poles (38.8452, 7.3482) (38.8452, 7.7758) (39.5694, 8.3072) (40.1131, 8.3072) knots 0 0 0 1 2 2 2
  spline S62 degree 2 poles (40.1131, 8.3072) (40.385, 8.3072) (40.9238, 8.196) (41.1364, 8.1021) knots 0 0 0 1 2 2 2
  line L54 (41.1364, 8.1021) -> (41.1364, 7.4051)
  line L55 (41.1364, 7.4051) -> (41.0696, 7.4051)
  spline S63 degree 2 poles (41.0696, 7.4051) (40.8991, 7.5509) (40.4097, 7.7511) (40.1527, 7.7511) knots 0 0 0 1 2 2 2
  spline S64 degree 2 poles (40.1527, 7.7511) (40.0513, 7.7511) (39.8931, 7.7215) (39.8042, 7.6819) knots 0 0 0 1 2 2 2
  spline S65 degree 2 poles (39.8042, 7.6819) (39.7325, 7.6498) (39.6287, 7.5213) (39.6287, 7.4422) knots 0 0 0 1 2 2 2
  spline S66 degree 2 poles (39.6287, 7.4422) (39.6287, 7.3235) (39.7943, 7.1876) (40.0316, 7.1332) knots 0 0 0 1 2 2 2
  spline S67 degree 2 poles (40.0316, 7.1332) (40.1848, 7.0986) (40.469, 7.0319) (40.6322, 6.975) knots 0 0 0 1 2 2 2
  spline S68 degree 2 poles (40.6322, 6.975) (40.9485, 6.8589) (41.2575, 6.4733) (41.2575, 6.1569) knots 0 0 0 1 2 2 2
  spline S69 degree 2 poles (41.2575, 6.1569) (41.2575, 5.7021) (40.5432, 5.1485) (39.9352, 5.1485) knots 0 0 0 1 2 2 2
  spline S70 degree 2 poles (44.0875, 6.1371) (44.0875, 5.9098) (43.9145, 5.5662) (43.7711, 5.4525) knots 0 0 0 1 2 2 2
  spline S71 degree 2 poles (43.7711, 5.4525) (43.5981, 5.3166) (43.1878, 5.2029) (42.869, 5.2029) knots 0 0 0 1 2 2 2
  line L56 (42.869, 5.2029) -> (41.6505, 5.2029)
  line L57 (41.6505, 5.2029) -> (41.6505, 8.2529)
  line L58 (41.6505, 8.2529) -> (42.7256, 8.2529)
  spline S72 degree 2 poles (42.7256, 8.2529) (43.0618, 8.2529) (43.4078, 8.201) (43.5586, 8.1194) knots 0 0 0 1 2 2 2
  spline S73 degree 2 poles (43.5586, 8.1194) (43.7242, 8.0329) (43.8848, 7.7363) (43.8848, 7.5435) knots 0 0 0 1 2 2 2
  spline S74 degree 2 poles (43.8848, 7.5435) (43.8848, 7.3211) (43.6624, 6.9726) (43.4647, 6.891) knots 0 0 0 1 2 2 2
  line L59 (43.4647, 6.891) -> (43.4647, 6.8762)
  spline S75 degree 2 poles (43.4647, 6.8762) (43.7489, 6.8168) (44.0875, 6.4486) (44.0875, 6.1371) knots 0 0 0 1 2 2 2
  spline S76 degree 2 poles (43.2966, 6.1495) (43.2966, 6.2929) (43.1829, 6.4535) (43.0692, 6.4955) knots 0 0 0 1 2 2 2
  spline S77 degree 2 poles (43.0692, 6.4955) (43, 6.5227) (42.7553, 6.5277) (42.5526, 6.5277) knots 0 0 0 1 2 2 2
  line L60 (42.5526, 6.5277) -> (42.4117, 6.5277)
  line L61 (42.4117, 6.5277) -> (42.4117, 5.759)
  line L62 (42.4117, 5.759) -> (42.4538, 5.759)
  spline S78 degree 2 poles (42.4538, 5.759) (42.7504, 5.759) (42.9778, 5.7664) (43.0964, 5.8183) knots 0 0 0 1 2 2 2
  spline S79 degree 2 poles (43.0964, 5.8183) (43.2002, 5.8653) (43.2966, 6.0383) (43.2966, 6.1495) knots 0 0 0 1 2 2 2
  spline S80 degree 2 poles (43.1063, 7.3927) (43.1063, 7.4669) (43.0297, 7.6226) (42.9506, 7.6572) knots 0 0 0 1 2 2 2
  spline S81 degree 2 poles (42.9506, 7.6572) (42.8764, 7.6918) (42.6688, 7.6967) (42.4637, 7.6967) knots 0 0 0 1 2 2 2
  line L63 (42.4637, 7.6967) -> (42.4117, 7.6967)
  line L64 (42.4117, 7.6967) -> (42.4117, 7.0492)
  line L65 (42.4117, 7.0492) -> (42.5081, 7.0492)
  spline S82 degree 2 poles (42.5081, 7.0492) (42.7034, 7.0492) (42.8616, 7.0566) (42.9456, 7.0961) knots 0 0 0 1 2 2 2
  spline S83 degree 2 poles (42.9456, 7.0961) (43.0371, 7.1406) (43.1063, 7.2914) (43.1063, 7.3927) knots 0 0 0 1 2 2 2
  point P0 (30.7841, 0)
  constraints: 4 other
extrude "Extrusão10" add sketch "Esboço11" along normal blind 0.8
